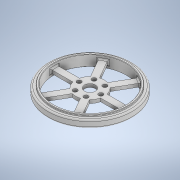
# Autodesk Inventor part: practiceWheel_09-10-19
Saved by Autodesk Inventor 2020 (Build 240168000, 168)
## iProperties
Created: 2019-09-10
Part Number: practiceWheel_09-10-19
Material: Generic
Document SubType Name: Modeling
Designer: dlr6513
Density: 1 g/cm^3
Appearance: Default
Author: dlr6513
Autodesk Inventor part; units mm, degrees
ref_plane "YZ Plane" through (0, 0, 0) normal (1, 0, 0) x (0, 1, 0)
ref_plane "XZ Plane" through (0, 0, 0) normal (0, 1, 0) x (-1, 0, 0)
ref_plane "XY Plane" through (0, 0, 0) normal (0, 0, 1) x (1, 0, 0)
sketch "Sketch1" plane through (0, 0, 0) normal (0, 1, 0) x (-1, 0, 0)
  circle A0 centre (51.4779, 117.7669) radius 35
  circle A1 centre (51.4779, 117.7669) radius 33
  circle A2 centre (51.4779, 117.7669) radius 38.5
  circle A3 centre (51.4779, 117.7669) radius 5
  circle A4 centre (51.4779, 117.7669) radius 13
  circle A5 centre (61.4779, 117.7669) radius 2
  circle A6 centre (56.4779, 126.4272) radius 2
  circle A7 centre (46.4779, 126.4272) radius 2
  circle A8 centre (41.4779, 117.7669) radius 2
  circle A9 centre (46.4779, 109.1067) radius 2
  circle A10 centre (56.4779, 109.1067) radius 2
  line L0 (84.3413, 114.7669) -> (64.127, 114.7669)
  line L1 (84.3413, 120.7669) -> (64.127, 120.7669)
  line L2 (65.3115, 147.7274) -> (55.2044, 130.2214)
  line L3 (70.5077, 144.7274) -> (60.4006, 127.2214)
  line L4 (32.4482, 144.7274) -> (42.5553, 127.2214)
  line L5 (37.6443, 147.7274) -> (47.7514, 130.2214)
  line L6 (18.6146, 114.7669) -> (38.8288, 114.7669)
  line L7 (18.6146, 120.7669) -> (38.8288, 120.7669)
  line L8 (37.6443, 87.8064) -> (47.7514, 105.3125)
  line L9 (32.4482, 90.8064) -> (42.5553, 108.3125)
  line L10 (70.5077, 90.8064) -> (60.4006, 108.3125)
  line L11 (65.3115, 87.8064) -> (55.2044, 105.3125)
  point P0 (0, 0)
  point P1 (84.4779, 114.7669)
  point P2 (61.4779, 114.7669)
  point P3 (84.4779, 120.7669)
  point P4 (61.4779, 120.7669)
  dimension "d0" = 70
  dimension "d1" = 66
  dimension "d2" = 77
  dimension "d3" = 10
  dimension "d4" = 26
  dimension "d6" = 4
  dimension "d9" = 360
  dimension "d14" = 360
  constraints: 24 end point, 11 centre point, 4 coincident, 4 point on circle, 50 other
  measures "d0" diameter of A0
  measures "d1" diameter of A1
  measures "d2" diameter of A2
  measures "d3" diameter of A3
  measures "d4" diameter of A4
  measures "d6" diameter of A5
extrude "Extrusion1" add sketch "Sketch1" along normal mid plane 7 contours A2
extrude "Extrusion2" add sketch "Sketch1" along normal mid plane 10 contours A0
extrude "Extrusion3" add sketch "Sketch1" along normal mid plane 3 contours A1 L0 A4 L1 | L3 A4 L2 A1 | A4 | A1 L11 A4 L10 | L5 A4 L4 A1 | A1 L9 A4 L8 | L7 A4 L6 A1
fillet "Fillet1" radius 1.397 2 edges at (-12.9779, 3.5, 117.7669) (-12.9779, -3.5, 117.7669)
fillet "Fillet2" radius 0.381 4 edges at (-16.4779, 5, 117.7669) (-16.4779, -5, 117.7669) (-18.4779, -5, 117.7669) (-18.4779, 5, 117.7669)
fillet "Fillet3" radius 1.27 37 edges at (-34.9779, -1.5, 146.3457) (-32.4482, 0.75, 144.7274) (-32.4482, -0.75, 144.7274) (-37.6443, 0.75, 147.7274) (-37.6443, -0.75, 147.7274) (-34.9779, 1.5, 146.3457) (-18.4779, 1.5, 117.7669) (-18.6146, 0.75, 120.7669) (-18.6146, -0.75, 120.7669) (-18.4779, -1.5, 117.7669) (-18.6146, 0.75, 114.7669) (-18.6146, -0.75, 114.7669) (-67.9779, -1.5, 146.3457) (-70.5077, 0.75, 144.7274) (-70.5077, -0.75, 144.7274) (-67.9779, 1.5, 146.3457) (-65.3115, 0.75, 147.7274) (-65.3115, -0.75, 147.7274) (-84.4437, -1.5, 116.2654) (-84.4437, -1.5, 119.2685) (-84.3413, 0.75, 114.7669) (-84.3413, -0.75, 114.7669) (-84.4437, 1.5, 116.2654) (-84.4437, 1.5, 119.2685) (-84.3413, 0.75, 120.7669) (-84.3413, -0.75, 120.7669) (-34.9779, 1.5, 89.1881) (-32.4482, 0.75, 90.8064) (-32.4482, -0.75, 90.8064) (-37.6443, 0.75, 87.8064) (-37.6443, -0.75, 87.8064) (-67.9779, 1.5, 89.1881) (-65.3115, 0.75, 87.8064) (-65.3115, -0.75, 87.8064) (-70.5077, 0.75, 90.8064) (-70.5077, -0.75, 90.8064) (-67.9779, -1.5, 89.1881)
body "Solid1"
